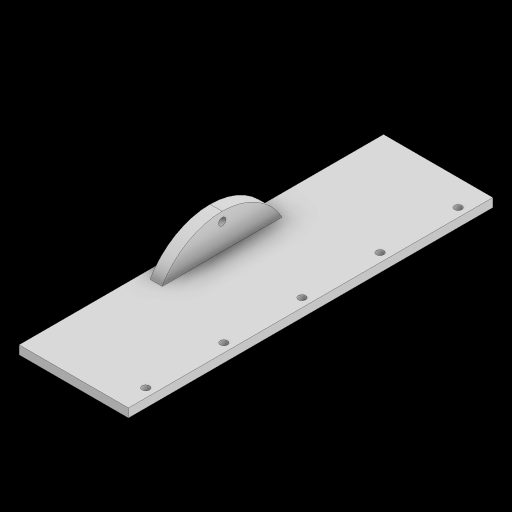
# Autodesk Inventor part: podstawa_sciana_front
Saved by Autodesk Inventor 2024.3 (Build 283343000, 343)
## iProperties
Created: 2025-10-10
Part Number: podstawa_sciana_front
Material: Ogólny
Document SubType Name: Modeling
Designer: User
Density: 1 g/cm^3
Appearance: Domyślna
Author: User
Autodesk Inventor part; units mm, degrees
ref_plane "YZ Plane" through (0, 0, 0) normal (1, 0, 0) x (0, 1, 0)
ref_plane "XZ Plane" through (0, 0, 0) normal (0, 1, 0) x (-1, 0, 0)
sketch "Szkic1" plane through (0, 0, 0) normal (0, 1, 0) x (-1, 0, 0)
  line L0 (-35, 105) -> (35, 105)
  line L1 (35, 105) -> (35, -105)
  line L2 (35, -105) -> (-35, -105)
  line L3 (-35, -105) -> (-35, 105)
  line L4 (-35, 105) -> (35, -105) construction
  line L5 (35, 105) -> (-35, -105) construction
  line L6 (-35, 105) -> (-25, 105)
  line L7 (-30, 105) -> (-30, 90)
  line L8 (35, 105) -> (28, 105)
  line L9 (28, 105) -> (28, -105)
  line L10 (35, -105) -> (28, -105)
  circle A0 centre (-30, 90) radius 2.15
  circle A1 centre (-30, 45) radius 2.15
  circle A2 centre (-30, 0) radius 2.15
  circle A3 centre (-30, -45) radius 2.15
  circle A4 centre (-30, -90) radius 2.15
  point P0 (0, 0)
  dimension "d0" = 70
  dimension "d1" = 210
  dimension "d2" = 10
  dimension "d3" = 15
  dimension "d4" = 7
  dimension "d5" = 4.3
  dimension "d8" = 45
  constraints: 22 end point, 5 centre point, 3 midpoint, 3 perpendicular, 3 point on line, 2 parallel, 2 vertical, 1 coincident, 1 horizontal, 8 other
  measures "d0" distance of L1.end L2.end
  measures "d1" distance of L0.end L1.end
  measures "d2" distance of L0.start L6.end
  measures "d3" distance of L7.start L7.end
  measures "d4" distance of L0.end L8.end
  measures "d5" diameter of A0
  measures "d8" distance of A0.centre A1.centre
extrude "Wyciągnięcie proste1" add sketch "Szkic1" along normal mid plane 5 contours L0 L9 L2 L3
ref_plane "Płaszczyzna konstrukcyjna1" through (-23, -2.5, 105) normal (-1, 0, 0) x (0, 0, 1)
sketch "Szkic2" plane through (-23, -2.5, 105) normal (-1, 0, 0) x (0, 0, 1)
  line L0 (0, 5) -> (-210, 5) projected
  line L1 (-210, 5) -> (0, 5)
  line L2 (-105, 5) -> (-105, 20)
  circle A0 centre (-105, 20) radius 2.15
  line L3 (-105, 22.15) -> (-105, 25.15)
  arc A1 (-105, 25.15) -> (-139.554, 5) centre (-104.8266, -14.8496) ccw
  arc A2 (-70.446, 5) -> (-105, 25.15) centre (-105.1734, -14.8496) ccw
  line L4 (-139.554, 5) -> (-70.446, 5)
  point P0 (-105, 2.5)
  point P1 (-70.446, 5)
  dimension "d17" = 4.3
  dimension "d16" = 15
  dimension "d18" = 3
  dimension "d19" = 40
  dimension "d20" = 40
  constraints: 8 end point, 4 point on circle, 2 centre point, 2 horizontal, 2 symmetric about line, 2 vertical, 1 coincident, 1 midpoint, 1 point on line, 1 vertical alignment, 3 other
  measures "d16" distance of L2.start L2.end
  measures "d18" distance of L3.start L3.end
  measures "d19" distance of L3.end L4.start
  measures "d20" radius of A1
extrude "Wyciągnięcie proste2" add sketch "Szkic2" against normal blind 7 contours L0 L2 A0 L3 A2 | L0 A1 L3 A0 L2
